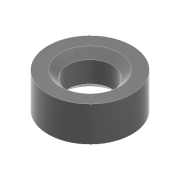
# Autodesk Inventor part: plastic M3 nut
Saved by Autodesk Inventor 2022 (Build 260153000, 153)
## iProperties
Created: 2024-09-01
Part Number: plastic M3 nut
Material: Generic
Document SubType Name: Modeling
Designer: david
Density: 1 g/cm^3
Appearance: Smooth - Black
Author: david
Autodesk Inventor part; units mm, degrees
ref_plane "YZ Plane" through (0, 0, 0) normal (1, 0, 0) x (0, 1, 0)
ref_plane "XZ Plane" through (0, 0, 0) normal (0, 1, 0) x (-1, 0, 0)
ref_plane "XY Plane" through (0, 0, 0) normal (0, 0, 1) x (1, 0, 0)
sketch "Sketch1" plane through (0, 0, 0) normal (0, 1, 0) x (-1, 0, 0)
  circle A0 centre (0, 0) radius 3
  dimension "d0" = 6
  constraints: 1 centre point, 1 coincident
  measures "d0" diameter of A0
extrude "Extrusion1" add sketch "Sketch1" along normal blind 2.5
sketch "Sketch2" plane through (0, 2.5, 0) normal (0, 1, 0) x (1, 0, 0)
  circle A0 centre (0, 0) radius 3 projected
  constraints: 1 coincident
hole "Hole1" at (0, 2.5, 0) direction (0, -1, 0) diameter 3.2 end through all
chamfer "Chamfer1" distance 0.5 angle 45 2 edges at (0, 2.5, -1.6) (0, 0, -1.6)
body "Solid1"
